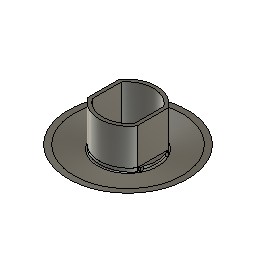
lock_shim (Autodesk Fusion 360 design; units mm, degrees)
Autodesk Fusion 360 part; units mm, degrees
sketch "Sketch1" plane through (0, 0, 0) normal (0, 0, 1) x (1, 0, 0) in component "Component"
  line L0 (0, 0) -> (0, 12)
  line L1 (19, 0) -> (19, 12)
  arc A0 (19, 12) -> (0, 12) centre (9.5, 5.5) ccw
  arc A1 (0, 0) -> (19, 0) centre (9.5, 6.5) ccw
  dimension "d1" = 12
  dimension "d2" = 12
  constraint coincident L0.start A1.start
  constraint vertical L0
  constraint vertical L1
  measures "d1" distance of L0.start L0.end
  measures "d2" distance of L1.end L1.start
extrude "Extrude1" add sketch "Sketch1" along normal blind 14 makes body 1 in component "Component"
sketch "Sketch2" plane through (0, 0, 14) normal (0, 0, 1) x (-1, 0, 0) in component "Component"
  arc A0 (0, 0) -> (-19, 0) centre (-9.5, -6.5) ccw
  line L0 (-19, 0) -> (-19, -12)
  arc A1 (-19, -12) -> (0, -12) centre (-9.5, -5.5) ccw
  line L1 (0, -12) -> (0, 0)
  line L2 (-1.3, -11.5846) -> (-1.3, -0.4155)
  arc A2 (-1.3, -0.4155) -> (-17.7, -0.4155) centre (-9.5, -6.5) ccw
  line L3 (-17.7, -0.4155) -> (-17.7, -11.5846)
  arc A3 (-17.7, -11.5846) -> (-1.3, -11.5846) centre (-9.5, -5.5) ccw
  dimension "d5" = -1.3
extrude "Extrude2" cut sketch "Sketch2" against normal blind 14 contours L2 A2 L3 A3 bodies 1 in component "Component"
sketch "Sketch2 (2)" plane through (0, 0, 0) normal (1, 0, 0) x (0, 1, 0) in component "Component'"
  line L0 (-9.8, 0) -> (-9.8, -2.9355)
  line L1 (-11, 0) -> (-11, -0.9648)
  line L2 (-11, 0) -> (-9.8, 0)
  line L3 (-9.8, -2.9355) -> (-15.506, -2.9355)
  line L4 (-23, 0) -> (-20.8108, 0)
  line L5 (-16.0723, -2.8245) -> (-23, 0)
  line L6 (-20.8108, 0) -> (-11.578, -1.4587)
  arc A0 (-11.578, -1.4587) -> (-11, -0.9648) centre (-11.5, -0.9648) ccw
  arc A1 (-16.0723, -2.8245) -> (-15.506, -2.9355) centre (-15.506, -1.4355) ccw
  point P0 (-15.8, -2.9355)
  dimension "d12" = 6
  dimension "d14" = 2.1892
  dimension "d15" = 0.5
  dimension "d16" = 1.5
  constraint vertical L0
  constraint perpendicular L0 L2
  constraint perpendicular L0 L3
  constraint horizontal L4
  constraint tangent L1 A0
  constraint tangent L6 A0
  constraint coincident P0 L3
  constraint coincident P0 L5
  constraint tangent L3 A1
  constraint tangent L5 A1
  measures "d12" distance of L0.end P0
  measures "d14" distance of L4.start L4.end
  measures "d15" radius of A0
  measures "d16" radius of A1
revolve "Revolve1" add sketch "Sketch2 (2)" angle 360 about axis through (9.5, 6, 1.75) along (0, 0, 1) separate body sketch seen with x (1, 0, 0) y (0, 1, 0) z (0, 0, 1) at (9.5, 6, 0) makes body 2
sketch "Sketch1 (2)" plane through (0, 0, 0) normal (0, 0, -1) x (1, 0, 0)
  line L0 (1.3, -11.5846) -> (1.3, -0.4155)
  arc A0 (17.7, -0.4155) -> (1.3, -0.4155) centre (9.5, -6.5) ccw
  line L1 (17.7, -0.4155) -> (17.7, -11.5846)
  arc A1 (1.3, -11.5846) -> (17.7, -11.5846) centre (9.5, -5.5) ccw
  arc A2 (19, 0) -> (0, 0) centre (9.5, -6.5) ccw
  line L2 (0, 0) -> (0, -12)
  arc A3 (0, -12) -> (19, -12) centre (9.5, -5.5) ccw
  line L3 (19, -12) -> (19, 0)
extrude "Extrude1'" add sketch "Sketch1 (2)" along normal blind 2.93 bodies 2
extrude "Extrude2'" add 1 faces at (17.7, 7.7889, -1.9533) along direction (1, 0, 0) blind 2 on bodies 2 bodies 2
extrude "Extrude3" add 1 faces at (1.3, 7.7889, -1.9533) along direction (-1, 0, 0) blind 2 on bodies 2 bodies 2
revolve "Revolve1'" [rolled back] along angle 360 in component "Component'"
extrude "Extrude3'" [rolled back] along distance 3 taper angle 0 in component "Component"
component "Component" placed x (1, 0, 0) y (0, 1, 0) z (0, 0, 1) at (0, 0, 0)
component "Component'" placed x (1, 0, 0) y (0, 1, 0) z (0, 0, 1) at (9.5, 6, 0)
